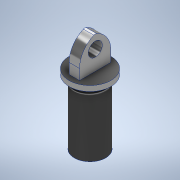
# Autodesk Inventor part: Part1
Saved by Autodesk Inventor 2020 (Build 240168000, 168)
## iProperties
Created: 2021-05-18
Part Number: Part1
Material: Aluminum 6061
Document SubType Name: Modeling
Designer: Andrew
Density: 2.7 g/cm^3
Appearance: Aluminum - Flat
Mass: 444.209 g
Surface Area: 295.699 cm^2
Volume: 164.522 cm^3
Author: Andrew
Autodesk Inventor part; units mm, degrees
ref_plane "YZ Plane" through (0, 0, 0) normal (1, 0, 0) x (0, 1, 0)
ref_plane "XZ Plane" through (0, 0, 0) normal (0, 1, 0) x (-1, 0, 0)
ref_plane "XY Plane" through (0, 0, 0) normal (0, 0, 1) x (1, 0, 0)
sketch "Sketch1" plane through (0, 0, 0) normal (1, 0, 0) x (0, 1, 0)
  line L0 (0, 0) -> (100, 0)
  line L1 (100, 0) -> (100, -30)
  line L2 (100, -30) -> (92.5, -30)
  line L3 (92.5, -30) -> (92.5, -22.4)
  line L4 (92.5, -22.4) -> (0, -22.4)
  line L5 (0, -22.4) -> (0, 0)
  line L6 (100, 0) -> (100, -22.5)
  line L7 (100, -22.5) -> (115, -22.5)
  line L8 (100, 0) -> (100, 22.5)
  line L9 (100, 22.5) -> (115, 22.5)
  circle A0 centre (127.721, -0.0575) radius 10
  arc A1 (146.8198, 0) -> (115, 22.5) centre (115, -11.25) ccw
  arc A2 (115, -22.5) -> (146.8198, 0) centre (115, 11.25) ccw
  dimension "d0" = 100
  dimension "d1" = 30
  dimension "d2" = 7.5
  dimension "d3" = 7.6
  dimension "d9" = 22.5
  dimension "d10" = 15
  dimension "d11" = 22.5
  dimension "d15" = 20
  dimension "d26" = 33.75
  dimension "d27" = 33.75
  constraints: 20 end point, 4 perpendicular, 4 point on circle, 3 centre point, 3 horizontal, 2 tangent, 2 vertical, 1 point on line
  measures "d0" distance of L0.start L0.end
  measures "d1" distance of L0.end L1.end
  measures "d2" distance of L1.end L2.end
  measures "d3" distance of L2.end L3.end
  measures "d9" distance of L0.end L6.end
  measures "d10" distance of L7.end L6.end
  measures "d11" distance of L0.end L8.end
  measures "d15" diameter of A0
  measures "d26" radius of A2
  measures "d27" radius of A1
revolve "Revolution1" add sketch "Sketch1" angle 360 about axis through (0, 0, 0) along (0, 1, 0) contours L0 L1 L2 L3 L4 L5
extrude "Extrusion1" add sketch "Sketch1" along normal mid plane 15 contours L8 L9 A1 A2 L7 L1
fillet "Fillet1" radius 5 1 edges at (0, 146.8198, 0)
thread "Thread1" size "M45x4.5" class "6g" standard "ANSI Metric M Profile" length 10
sketch "Sketch2" plane through (0, 0, 0) normal (0, -1, 0) x (1, 0, 0)
  circle A0 centre (0, 0) radius 10
  dimension "d23" = 20
  constraints: 1 centre point, 1 coincident
  measures "d23" diameter of A0
extrude "Extrusion2" cut sketch "Sketch2" against normal blind 75
body "Solid1"
